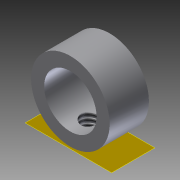
# Autodesk Inventor part: Jig_Aligner_Sleeve
Saved by Autodesk Inventor 2011 SP2 (Build 150309200, 309)
## iProperties
Created: 2012-02-29
Part Number: Jig_Aligner_Sleeve
Document SubType Name: Modeling
Designer: sungwook
Density: 1 g/cm^3
Author: sungwook
Autodesk Inventor part; units mm, degrees
ref_plane "YZ Plane" through (0, 0, 0) normal (1, 0, 0) x (0, 1, 0)
ref_plane "XY Plane" through (0, 0, 0) normal (0, 0, 1) x (1, 0, 0)
sketch "Sketch1" plane through (0, 0, 0) normal (0, 0, 1) x (1, 0, 0)
  circle A0 centre (0, 0) radius 3.81
  dimension "d0" = 7.62
  constraints: 1 centre point, 1 coincident
  measures "d0" diameter of A0
extrude "Extrusion1" add sketch "Sketch1" along normal blind 3.81
hole "Hole1" at (0, 0, 0) direction (0, 0, 1) diameter 5.08 end through all
ref_plane "Work Plane1" through (0, 0, 3.81) normal (0, 0, -1) x (-1, 0, 0)
ref_plane "Work Plane2" through (0, -3.81, 0) normal (0, -1, 0) x (1, 0, 0)
sketch "Sketch2" plane through (0, -3.81, 0) normal (0, -1, 0) x (1, 0, 0)
  point P0 (0, 0)
sketch "Sketch3" plane through (0, -3.81, 0) normal (0, -1, 0) x (1, 0, 0)
  line L0 (-3.81, 3.81) -> (3.81, 3.81) projected
  line L1 (-3.81, 0) -> (3.81, 0) projected
  line L2 (0, -0.762) -> (0, 4.572) projected
  line L3 (0, 3.81) -> (0, 0)
  point P0 (0, 1.905)
  dimension "d15" = 1.905
  constraints: 2 end point, 2 midpoint, 1 collinear, 1 point on line
  measures "d15" distance from line of point (0, 1.905) L0
hole "Hole2" at (0, -3.81, 1.905) direction (0, 1, 0) diameter 1.7018 depth 3.81
equation "\"d12\" = -d1"
equation "\"d1\" = 3.81"
body "Solid1"
